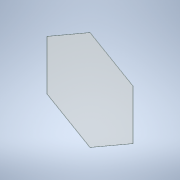
# Autodesk Inventor part: Top
Saved by Autodesk Inventor 2020.3 (Build 243373000, 373)
## iProperties
Created: 2020-07-07
Part Number: Top
Material: Glass
Document SubType Name: Modeling
Designer: Bruno
Density: 2.18 g/cm^3
Appearance: Clear
Author: Bruno
Autodesk Inventor part; units mm, degrees
ref_plane "YZ Plane" through (0, 0, 0) normal (1, 0, 0) x (0, 1, 0)
ref_plane "XZ Plane" through (0, 0, 0) normal (0, 1, 0) x (-1, 0, 0)
ref_plane "Work Plane1" through (0, 0, 0) normal (0, 0, 1) x (1, 0, 0)
sketch "Sketch1" plane through (0, 0, 0) normal (0, 0, 1) x (1, 0, 0)
  line L0 (500, -288.6751) -> (0, -577.3503)
  line L1 (0, -577.3503) -> (-500, -288.6751)
  line L2 (-500, -288.6751) -> (-500, 288.6751)
  line L3 (-500, 288.6751) -> (0, 577.3503)
  line L4 (0, 577.3503) -> (500, 288.6751)
  line L5 (500, 288.6751) -> (500, -288.6751)
  point P0 (0, 0)
  point P1 (0, 0)
  point P2 (0, 0)
  dimension "d1" = 500
  constraints: 12 end point, 2 coincident, 1 vertical, 13 other
  measures "d1" distance from line of point (0, 0) L5
extrude "Extrusion1" add sketch "Sketch1" along normal blind 4
body "Solid1"
